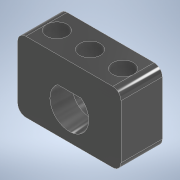
# Autodesk Inventor part: pendulum_adapter
Saved by Autodesk Inventor 2021 (Build 250183000, 183)
## iProperties
Created: 2022-06-20
Part Number: pendulum_adapter
Material: ABS Plastic
Document SubType Name: Modeling
Designer: lenna
Density: 1.06 g/cm^3
Appearance: Smooth - White
Mass: 3.40151 g
Surface Area: 22.0772 cm^2
Volume: 3.20897 cm^3
Author: lenna
Autodesk Inventor part; units mm, degrees
note: some values were not read from the file. Chosen so that the rebuilt part matches the saved one: direction of "Hole1"; direction of "Hole2".
ref_plane "YZ Plane" through (0, 0, 0) normal (1, 0, 0) x (0, 1, 0)
ref_plane "XZ Plane" through (0, 0, 0) normal (0, 1, 0) x (-1, 0, 0)
ref_plane "XY Plane" through (0, 0, 0) normal (0, 0, 1) x (1, 0, 0)
sketch "Sketch1" plane through (0, 0, 0) normal (0, 0, 1) x (1, 0, 0)
  circle A0 centre (0, 0) radius 4.25
  line L0 (-2.4109, 3.5) -> (2.4109, 3.5)
  line L1 (-12.5, 10) -> (12.5, 10)
  line L2 (12.5, 10) -> (12.5, -7)
  line L3 (12.5, -7) -> (-12.5, -7)
  line L4 (-12.5, -7) -> (-12.5, 10)
  dimension "d0" = 8.5
  dimension "d1" = 3.5
  dimension "d2" = 25
  dimension "d3" = 12.5
  dimension "d4" = 17
  dimension "d5" = 10
  constraints: 10 end point, 2 horizontal, 2 parallel, 2 point on circle, 1 centre point, 1 coincident, 1 perpendicular
  measures "d0" diameter of A0
  measures "d1" distance from line of point (0, 0) L0
  measures "d2" distance between parallel lines of L2 L4
  measures "d3" distance from line of point (0, 0) L4
  measures "d4" distance between parallel lines of L3 L1
  measures "d5" distance from line of point (0, 0) L1
extrude "Extrusion1" add sketch "Sketch1" along normal blind 10 contours L0 A0 | L1 L2 L3 L4 picked at (-0.1705, 3.7397)
sketch "Sketch2" plane through (-12.5, 10, 0) normal (0, 1, 0) x (1, 0, 0)
  line L0 (25, -10) -> (0, -10) projected
  line L1 (25, 0) -> (0, 0) projected
  line L2 (0, 0) -> (0, -10) projected
  point P0 (12.5, 0)
  point P1 (4.5, -5)
  dimension "d8" = 10
  dimension "d9" = 5
  dimension "d18" = 8
  measures "d8" distance between parallel lines of L0 L1
  measures "d9" distance from line of L1 point (4.5, -5)
  measures "d18" horizontal distance of point (12.5, 0) point (4.5, -5)
hole "Hole1" at (-8, 10, 5) direction (0, -1, 0) diameter 3.5 depth 17 counterbore diameter 5 counterbore depth 5
mirror "Mirror1" about plane through (0, 0, 0) normal (1, 0, 0) of "Hole1"
sketch "Sketch3" plane through (-12.5, 10, 0) normal (0, 1, 0) x (1, 0, 0)
  line L0 (25, -10) -> (0, -10) projected
  line L1 (25, 0) -> (0, 0) projected
  line L2 (25, 0) -> (25, -10) projected
  line L3 (0, 0) -> (0, -10) projected
  point P0 (12.5, 0)
  point P1 (12.5, -5)
  dimension "d19" = 10
  dimension "d20" = 5
  dimension "d21" = 25
  dimension "d22" = 12.5
  measures "d19" distance between parallel lines of L0 L1
  measures "d20" distance from line of L1 point (12.5, -5)
  measures "d21" distance between parallel lines of L2 L3
  measures "d22" distance from line of L3 point (12.5, -5)
hole "Hole2" at (0, 10, 5) direction (0, -1, 0) diameter 5 end up to surface
fillet "Fillet1" radius 2 4 edges at (-12.5, 10, 5) (12.5, 10, 5) (12.5, -7, 5) (-12.5, -7, 5)
chamfer "Chamfer1" distance 5 angle 5 1 edges at (0, -4.25, 10)
chamfer "Chamfer2" distance 2.5 angle 5 1 edges at (0, 3.5, 10) measured on face at (0, 3.5, 9.1667)
equation "\"d3\" = 0.5 * d2"
equation "\"d9\" = 0.5 * d8"
equation "\"d20\" = 0.5 * d19"
equation "\"d22\" = 0.5 * d21"
body "Solid1"
